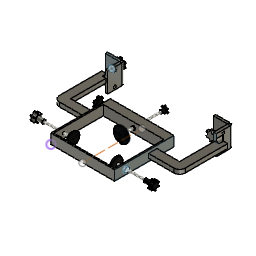
Wheelchair_Bracket (Autodesk Fusion 360 design; units mm, degrees)
Autodesk Fusion 360 part; units mm, degrees
note: some values were not read from the file. Chosen so that the rebuilt part matches the saved one: which face or edge a step refers to; how an offset face is resized.
sketch "Schizzo1" plane through (0, 0, 0) normal (0, 0, 1) x (1, 0, 0)
  line L0 (0, 0) -> (225, 0)
  line L1 (225, 0) -> (225, 210)
  line L2 (225, 210) -> (0, 210)
  line L3 (0, 210) -> (0, 0)
  line L4 (5, 180) -> (5, 5)
  line L5 (5, 5) -> (220, 5)
  line L6 (220, 5) -> (220, 180)
  line L7 (0, 150) -> (-75, 150)
  line L8 (0, 120) -> (-110, 120)
  line L9 (-110, 120) -> (-110, 290)
  line L10 (-110, 290) -> (-80, 290)
  line L11 (-80, 290) -> (-80, 150)
  line L12 (-80, 150) -> (-75, 150)
  line L13 (335, 120) -> (335, 290)
  line L14 (305, 290) -> (305, 150)
  line L15 (335, 290) -> (305, 290)
  line L16 (225, 120) -> (335, 120)
  line L17 (225, 150) -> (300, 150)
  line L18 (300, 150) -> (305, 150)
  line L19 (5, 180) -> (220, 180)
  dimension "d1" = 225
  dimension "d2" = 210
  dimension "d5" = 30
  dimension "d8" = 30
  constraint horizontal L0
  constraint vertical L1
  constraint horizontal L2
  constraint vertical L3
  constraint coincident L0.start L3.end
  constraint coincident L3 L7.start
  constraint perpendicular L3 L7
  constraint coincident L3 L8.start
  constraint perpendicular L3 L8
  constraint perpendicular L8 L9
  constraint perpendicular L9 L10
  constraint perpendicular L7 L11
  constraint perpendicular L11 L12
  constraint perpendicular L1 L19
  constraint parallel L3 L4
  constraint parallel L0 L5
  constraint parallel L1 L6
  measures "d1" distance of L0.start L0.end
  measures "d2" distance of L0.start L2.end
  measures "d5" distance of L7 L8
  measures "d8" distance of L2 L19
extrude "Estrusione1" add sketch "Schizzo1" along normal blind 35 contours L0 L1 L2 L3 makes body 1
extrude "Estrusione2" add sketch "Schizzo1" along normal blind 25 contours L3 L7 L8 L9 L10 L11 L12 | L1 L13 L14 L15 L16 L17 L18 bodies 1
extrude "Estrusione3" cut sketch "Schizzo1" along normal blind 10 contours L3 L7 L8 L9 L10 L11 L12 | L1 L13 L14 L15 L16 L17 L18 bodies 1
sketch "Schizzo2" plane through (0, 180, 0) normal (0, -1, 0) x (1, 0, 0)
  line L0 (5, 0) -> (220, 0)
  line L1 (220, 0) -> (220, 35)
  line L2 (220, 35) -> (5, 35)
  line L3 (5, 35) -> (5, 0)
sketch "Schizzo3" plane through (0, 210, 0) normal (0, 1, 0) x (-1, 0, 0)
  line L0 (-225, 0) -> (0, 0)
  line L1 (0, 0) -> (0, 35)
  line L2 (0, 35) -> (-225, 35)
  line L3 (-225, 35) -> (-225, 0)
  circle A0 centre (-112.5, 17.5615) radius 4
  dimension "d17" = 8
  dimension "d18" = 112.5
  measures "d17" diameter of A0
  measures "d18" distance of L3 A0.centre
extrude "Estrusione5" cut sketch "Schizzo3" along normal mid plane 100 contours A0 bodies 1
extrude "Estrusione8" add sketch "Schizzo3" along normal mid plane 140 separate body contours A0 makes body 2
thread "Filettatura2" "ISO Metric profile 8.0 M8x1.25 6g" major diameter 7.866 minor diameter 6.4455 pitch 1.25 angle 60 resizes the face on face at (108.5199, 256.6667, 17.1632) on bodies 2
sketch "Schizzo4" plane through (0, 280, 0) normal (0, 1, 0) x (-1, 0, 0)
  circle A0 centre (-112.5, 17.5615) radius 3.933
  circle A1 centre (-112.5, 17.5615) radius 6.5
  dimension "d29" = 13
  constraint concentric A0 A1
  measures "d29" diameter of A1
extrude "Estrusione9" add sketch "Schizzo4" along normal blind 8 contours A0 | A1 bodies 2
extrude "Estrusione10" add 1 faces at (106.8945, 280, 17.0432) along direction (0, -1, 0) blind 3 on bodies 2 bodies 2
sketch "Schizzo6" plane through (0, 288, 0) normal (0, 1, 0) x (-1, 0, 0)
  circle A0 centre (-112.5, 17.5615) radius 6.5
  circle A1 centre (-112.5, 17.5615) radius 12.5
  circle A2 centre (-125, 17.5615) radius 6.1387
  circle A3 centre (-118.75, 6.7362) radius 6.1387
  circle A4 centre (-106.25, 6.7362) radius 6.1387
  circle A5 centre (-100, 17.5615) radius 6.1387
  circle A6 centre (-106.25, 28.3868) radius 6.1387
  circle A7 centre (-118.75, 28.3868) radius 6.1387
  dimension "d38" = 25
  dimension "d40" = 360
  constraint concentric A0 A1
  constraint coincident A1 A2.centre
  measures "d38" diameter of A1
extrude "Estrusione12" add sketch "Schizzo6" along normal blind 6 contours A0 A2 A3 A4 A5 A6 A7 | A0 A1 A5 A6 | A0 A1 A4 A5 | A0 A1 A6 A7 | A0 A1 A3 A4 | A0 A1 A2 A7 | A0 A1 A2 A3 bodies 2
fillet "Raccordo3" radius 20 1 edges at (-110, 120, 17.5) on bodies 1
fillet "Raccordo4" radius 20 1 edges at (335, 120, 17.5) on bodies 1
sketch "Schizzo7" plane through (0, 0, 0) normal (0, 0, 1) x (1, 0, 0)
sketch "Schizzo8" plane through (0, 140, 0) normal (0, -1, 0) x (1, 0, 0)
  circle A0 centre (112.5, 17.5615) radius 3.933
  circle A1 centre (112.5, 17.5615) radius 25
  dimension "d51" = 50
  constraint concentric A0 A1
  measures "d51" diameter of A1
extrude "Estrusione13" add sketch "Schizzo8" along normal blind 5 draft 20 separate body makes body 3
sketch "Schizzo9" plane through (225, 0, 0) normal (1, 0, 0) x (0, 1, 0)
  line L0 (0, 0) -> (210, 0)
  line L1 (210, 0) -> (210, 35)
  line L2 (210, 35) -> (0, 35)
  line L3 (0, 35) -> (0, 0)
  line L4 (150, 10) -> (120, 10)
  line L5 (120, 10) -> (120, 25)
  line L6 (120, 25) -> (150, 25)
  line L7 (150, 25) -> (150, 10)
  circle A0 centre (40, 17.5) radius 4
  line L8 (0, 0) -> (210, 0)
  dimension "d54" = 8
  dimension "d55" = 40
  dimension "d56" = 17.5
  measures "d54" diameter of A0
  measures "d55" distance of L3 A0.centre
  measures "d56" distance of A0.centre L8
extrude "Estrusione15" add sketch "Schizzo9" along normal blind 80 separate body contours A0 makes body 4
extrude "Estrusione23" add sketch "Schizzo9" against normal blind 30 contours A0 bodies 4
thread "Filettatura4" "ISO Metric profile 8.0 M8x1.25 6g" major diameter 7.866 minor diameter 6.4455 pitch 1.25 angle 60 resizes the face on face at (278.3333, 43.995, 17.3006) on bodies 4
sketch "Schizzo13" plane through (195, 0, 0) normal (-1, 0, 0) x (0, -1, 0)
  circle A0 centre (-40, 17.5) radius 3.933
  circle A1 centre (-40, 17.5) radius 20
  dimension "d83" = 40
  constraint concentric A0 A1
  measures "d83" diameter of A1
extrude "Estrusione24" add sketch "Schizzo13" along normal blind 5 draft 25 separate body makes body 5
sketch "Schizzo14" plane through (305, 0, 0) normal (1, 0, 0) x (0, 1, 0)
  circle A0 centre (40, 17.5) radius 3.933
  circle A1 centre (40, 17.5) radius 7.5
  dimension "d86" = 15
  constraint concentric A0 A1
  measures "d86" diameter of A1
extrude "Estrusione25" add sketch "Schizzo14" along normal mid plane 20 bodies 4
extrude "Estrusione26" add 1 faces at (305, 38.9168, 16.3707) along direction (1, 0, 0) blind 10 on bodies 4 bodies 4
sketch "Schizzo15" plane through (0, 0, 0) normal (0, 0, 1) x (1, 0, 0)
sketch "Schizzo16" plane through (315, 0, 0) normal (1, 0, 0) x (0, 1, 0)
  circle A0 centre (40, 17.5) radius 7.5
  circle A1 centre (40, 17.5) radius 15
  circle A2 centre (25, 17.5) radius 6
  circle A3 centre (32.5, 4.5096) radius 6
  circle A4 centre (47.5, 4.5096) radius 6
  circle A5 centre (55, 17.5) radius 6
  circle A6 centre (47.5, 30.4904) radius 6
  circle A7 centre (32.5, 30.4904) radius 6
  dimension "d91" = 30
  dimension "d92" = 12
  dimension "d94" = 360
  constraint concentric A0 A1
  constraint coincident A1 A2.centre
  measures "d91" diameter of A1
  measures "d92" diameter of A2
extrude "Estrusione27" add sketch "Schizzo16" along normal blind 15 contours A0 | A1 A2 A3 A4 A5 A6 A7 bodies 4
sketch "Schizzo17" plane through (0, 0, 0) normal (0, 0, 1) x (1, 0, 0)
  line L0 (112.5, 0) -> (112.5, 210) construction
  dimension "d97" = 112.5
  constraint vertical L0
  measures "d97" distance of L0.start origin
ref_plane "Piano di lavoro1" through (115, 105, 17.5) normal (1, 0, 0) x (0, 1, 0)
mirror "Specchio1" about plane through (115, 105, 17.5) normal (1, 0, 0) of bodies 4 5 makes body 6 at (-31.6667, 43.9281, 17.304) makes body 7 at (40, 24.6676, 16.311)
sketch "Schizzo18" plane through (305, 0, 0) normal (-1, 0, 0) x (0, -1, 0)
  line L0 (-290, 10) -> (-150, 10)
  line L1 (-150, 10) -> (-150, 25)
  line L2 (-150, 25) -> (-290, 25)
  line L3 (-290, 25) -> (-290, 10)
  line L4 (-275, -20) -> (-325, -20)
  line L5 (-325, -20) -> (-325, 50)
  line L6 (-325, 50) -> (-275, 50)
  line L7 (-275, 50) -> (-275, -20)
  constraint horizontal L4
  constraint vertical L5
  constraint horizontal L6
  constraint vertical L7
extrude "Estrusione28" add sketch "Schizzo18" along normal blind 5 contours L0 L2 L3 L7 | L0 L2 L3 L4 L5 L6 L7 bodies 1
extrude "Estrusione29" add 1 faces at (305, 313.3333, 13.3333) along direction (1, 0, 0) blind 5 on bodies 1 bodies 1
sketch "Schizzo19" plane through (300, 0, 0) normal (-1, 0, 0) x (0, -1, 0)
  line L0 (-275, 50) -> (-325, 50)
  line L1 (-325, 50) -> (-325, -20)
  line L2 (-325, -20) -> (-275, -20)
  line L3 (-275, -20) -> (-275, 50)
  circle A0 centre (-300, -10) radius 5
  circle A1 centre (-300, 40) radius 5
  dimension "d104" = 10
  dimension "d105" = 10
  measures "d104" diameter of A0
  measures "d105" diameter of A1
extrude "Estrusione30" cut sketch "Schizzo19" against normal blind 35 contours A0 | A1 bodies 1
fillet "Raccordo5" radius 10 3 edges at (310, 282.5, 10) (310, 290, 17.5) (310, 282.5, 25) on bodies 1
sketch "Schizzo1 (2)" plane through (0, 275, 0) normal (0, -1, 0) x (1, 0, 0) in component "Component"
  line L0 (310, 50) -> (300, 50)
  line L1 (300, 50) -> (300, -20)
  line L2 (300, -20) -> (310, -20)
  line L3 (310, -20) -> (310, 0)
  arc A0 (320, 10) -> (310, 0) centre (320, 0) ccw
  line L4 (320, 10) -> (305, 10)
  line L5 (305, 10) -> (305, 25)
  line L6 (305, 25) -> (320, 25)
  arc A1 (310, 35) -> (320, 25) centre (320, 35) ccw
  line L7 (310, 35) -> (310, 50)
sketch "Schizzo3 (2)" plane through (0, 325, 0) normal (0, 1, 0) x (-1, 0, 0) in component "Component"
  line L0 (-310, -20) -> (-300, -20)
  line L1 (-300, -20) -> (-300, 50)
  line L2 (-300, 50) -> (-310, 50)
  line L3 (-310, 50) -> (-310, -20)
sketch "Schizzo20" plane through (0, 0, 0) normal (0, 0, 1) x (1, 0, 0)
  circle A0 centre (305, 329) radius 4
  line L0 (300, 325) -> (310, 325)
  dimension "d112" = 8
  constraint tangent A0 L0
  measures "d112" diameter of A0
extrude "Estrusione31" add sketch "Schizzo20" along normal blind 50 separate body makes body 8
extrude "Estrusione32" add 1 faces at (305.2524, 327.9512, 0) along direction (0, 0, -1) blind 20 on bodies 8 bodies 8 4 5 6 7 1
sketch "Schizzo21" plane through (0, 325, 0) normal (0, 1, 0) x (-1, 0, 0)
  line L0 (-300, -20) -> (-250, -20)
  line L1 (-250, -20) -> (-250, 50)
  line L2 (-250, 50) -> (-300, 50)
  line L3 (-300, 50) -> (-300, -20)
  constraint horizontal L0
  constraint vertical L1
  constraint horizontal L2
  constraint vertical L3
extrude "Estrusione33" add sketch "Schizzo21" along normal blind 5 separate body makes body 9
extrude "Estrusione36" add 1 faces at (283.3333, 330, 26.6667) along direction (0, 1, 0) blind 3 on bodies 9 bodies 9
sketch "Schizzo22" plane through (0, 333, 0) normal (0, 1, 0) x (-1, 0, 0)
  line L0 (-300, 50) -> (-300, -20)
  line L1 (-300, -20) -> (-250, -20)
  line L2 (-250, -20) -> (-250, 50)
  line L3 (-250, 50) -> (-300, 50)
  circle A0 centre (-275, 17.5) radius 4
  dimension "d129" = 8
  dimension "d130" = 25
  dimension "d131" = 32.5
  measures "d129" diameter of A0
  measures "d130" distance of L2 A0.centre
  measures "d131" distance of L3 A0.centre
extrude "Estrusione37" add sketch "Schizzo22" along normal blind 20 and the other way blind 25 contours A0 bodies 9
thread "Filettatura5" "ISO Metric profile 8.0 M8x1.25 6g" major diameter 7.866 minor diameter 6.4455 pitch 1.25 angle 60 resizes the face on face at (272.665, 313.6667, 20.7478) on bodies 9
thread "Filettatura6" "ISO Metric profile 8.0 M8x1.25 6g" major diameter 7.866 minor diameter 6.4455 pitch 1.25 angle 60 resizes the face on face at (272.665, 339.6667, 20.7478) on bodies 9
sketch "Schizzo24" plane through (0, 308, 0) normal (0, -1, 0) x (1, 0, 0)
  circle A0 centre (275, 17.5) radius 3.933
  circle A1 centre (275, 17.5) radius 7.5
  dimension "d137" = 15
  constraint concentric A0 A1
  measures "d137" diameter of A1
extrude "Estrusione38" add sketch "Schizzo24" along normal mid plane 20 bodies 9
extrude "Estrusione39" add 1 faces at (276.5445, 308, 16.6083) along direction (0, -1, 0) blind 10 on bodies 9 bodies 9
sketch "Schizzo25" plane through (0, 298, 0) normal (0, -1, 0) x (1, 0, 0)
  circle A0 centre (275, 17.5) radius 7.5
  circle A1 centre (275, 17.5) radius 17.5
  circle A2 centre (257.5, 17.5) radius 6
  circle A3 centre (266.25, 2.3446) radius 6
  circle A4 centre (283.75, 2.3446) radius 6
  circle A5 centre (292.5, 17.5) radius 6
  circle A6 centre (283.75, 32.6554) radius 6
  circle A7 centre (266.25, 32.6554) radius 6
  dimension "d142" = 35
  dimension "d143" = 12
  dimension "d145" = 360
  constraint concentric A0 A1
  constraint coincident A1 A2.centre
  measures "d142" diameter of A1
  measures "d143" diameter of A2
extrude "Estrusione40" add sketch "Schizzo25" along normal blind 8 contours A0 | A1 A2 A3 A4 A5 A6 A7 bodies 9
extrude "Estrusione41" cut 1 faces at (277.6423, 318, 11.7874) along direction (0, -1, 0) blind 10 on bodies 9 bodies 9
sketch "Schizzo26" plane through (0, 333, 0) normal (0, 1, 0) x (-1, 0, 0)
  circle A0 centre (-275, 17.5) radius 3.933
  line L0 (-300, 50) -> (-300, -20)
  line L1 (-300, -20) -> (-250, -20)
  line L2 (-250, -20) -> (-250, 50)
  line L3 (-250, 50) -> (-300, 50)
  line L4 (-268.0719, 17.4702) -> (-271.5101, 23.485)
  line L5 (-271.5101, 23.485) -> (-278.4383, 23.5148)
  line L6 (-278.4383, 23.5148) -> (-281.9281, 17.5298)
  line L7 (-281.9281, 17.5298) -> (-278.4899, 11.515)
  line L8 (-278.4899, 11.515) -> (-271.5617, 11.4852)
  line L9 (-271.5617, 11.4852) -> (-268.0719, 17.4702)
  point P0 (-275, 17.5)
  dimension "d150" = 6
  constraint coincident P0 A0.centre
  measures "d150" distance of P0 L9
extrude "Estrusione42" add sketch "Schizzo26" along normal blind 2 separate body contours L4 L5 L6 L7 L8 L9 makes body 10
sketch "Schizzo27" plane through (0, 180, 0) normal (0, -1, 0) x (1, 0, 0)
  circle A0 centre (112.5, 17.5615) radius 4
  line L0 (5, 0) -> (220, 0)
  line L1 (220, 0) -> (220, 35)
  line L2 (220, 35) -> (5, 35)
  line L3 (5, 35) -> (5, 0)
  line L4 (119.4226, 17.8407) -> (115.7195, 23.6962)
  line L5 (115.7195, 23.6962) -> (108.7969, 23.417)
  line L6 (108.7969, 23.417) -> (105.5774, 17.2822)
  line L7 (105.5774, 17.2822) -> (109.2805, 11.4267)
  line L8 (109.2805, 11.4267) -> (116.2031, 11.706)
  line L9 (116.2031, 11.706) -> (119.4226, 17.8407)
  point P0 (112.5, 17.5615)
  dimension "d153" = 6
  constraint coincident P0 A0.centre
  measures "d153" distance of P0 L9
extrude "Estrusione43" add sketch "Schizzo27" along normal blind 2 separate body contours L4 L5 L6 L7 L8 L9 makes body 11
sketch "Schizzo28" plane through (225, 0, 0) normal (1, 0, 0) x (0, 1, 0)
  line L0 (0, 0) -> (210, 0)
  line L1 (210, 0) -> (210, 35)
  line L2 (210, 35) -> (0, 35)
  line L3 (0, 35) -> (0, 0)
  line L4 (150, 10) -> (120, 10)
  line L5 (120, 10) -> (120, 25)
  line L6 (120, 25) -> (150, 25)
  line L7 (150, 25) -> (150, 10)
  line L8 (41.2349, 25.5706) -> (34.8128, 23.9335)
  line L9 (34.8128, 23.9335) -> (31.4294, 18.2349)
  line L10 (31.4294, 18.2349) -> (33.0665, 11.8128)
  line L11 (33.0665, 11.8128) -> (38.7651, 8.4294)
  line L12 (38.7651, 8.4294) -> (45.1872, 10.0665)
  line L13 (45.1872, 10.0665) -> (48.5706, 15.7651)
  line L14 (48.5706, 15.7651) -> (46.9335, 22.1872)
  line L15 (46.9335, 22.1872) -> (41.2349, 25.5706)
  point P0 (40, 17)
  dimension "d156" = 8
  measures "d156" distance of P0 L15
extrude "Estrusione44" add sketch "Schizzo28" along normal blind 4 separate body contours L8 L9 L10 L11 L12 L13 L14 L15 makes body 12
mirror "Specchio2" about plane through (115, 105, 17.5) normal (1, 0, 0) of bodies 12 makes body 13
mirror "Specchio3" about plane through (115, 105, 17.5) normal (1, 0, 0) of bodies 12 makes body 14
mirror "Specchio4" about plane through (115, 105, 17.5) normal (1, 0, 0) of bodies 12 makes body 15
extrude "Estrusione45" add 1 faces at (5, 39.5884, 14.1431) along direction (-1, 0, 0) blind 10 on bodies 15 bodies 15 7 11 12 6 8 13 14
sketch "Schizzo29" plane through (0, 0, 0) normal (0, 0, 1) x (1, 0, 0)
sketch "Schizzo30" plane through (0, 0, 0) normal (-1, 0, 0) x (0, -1, 0)
  line L0 (-41.2349, 25.5706) -> (-34.8128, 23.9335)
  line L1 (-34.8128, 23.9335) -> (-31.4294, 18.2349)
  line L2 (-31.4294, 18.2349) -> (-33.0665, 11.8128)
  line L3 (-33.0665, 11.8128) -> (-38.7651, 8.4294)
  line L4 (-38.7651, 8.4294) -> (-45.1872, 10.0665)
  line L5 (-45.1872, 10.0665) -> (-48.5706, 15.7651)
  line L6 (-48.5706, 15.7651) -> (-46.9335, 22.1872)
  line L7 (-46.9335, 22.1872) -> (-41.2349, 25.5706)
  line L8 (-120, 10) -> (-150, 10)
  line L9 (-150, 10) -> (-150, 25)
  line L10 (-150, 25) -> (-120, 25)
  line L11 (-120, 25) -> (-120, 10)
  line L12 (-210, 0) -> (0, 0)
  line L13 (0, 0) -> (0, 35)
  line L14 (0, 35) -> (-210, 35)
  line L15 (-210, 35) -> (-210, 0)
  circle A0 centre (-194.5679, 17.5) radius 4
  dimension "d169" = 8
  dimension "d170" = 17.5
  measures "d169" diameter of A0
  measures "d170" distance of L14 A0.centre
extrude "Estrusione46" add sketch "Schizzo30" along normal blind 20 and the other way blind 0 separate body contours A0 makes body 16
thread "Filettatura7" "ISO Metric profile 8.0 M8x1.25 6g" major diameter 7.866 minor diameter 6.4455 pitch 1.25 angle 60 resizes the face on face at (-13.3333, 197.6321, 20.0712) on bodies 16
sketch "Schizzo31" plane through (0, 0, 0) normal (-1, 0, 0) x (0, -1, 0)
  line L0 (-41.2349, 25.5706) -> (-34.8128, 23.9335)
  line L1 (-34.8128, 23.9335) -> (-31.4294, 18.2349)
  line L2 (-31.4294, 18.2349) -> (-33.0665, 11.8128)
  line L3 (-33.0665, 11.8128) -> (-38.7651, 8.4294)
  line L4 (-38.7651, 8.4294) -> (-45.1872, 10.0665)
  line L5 (-45.1872, 10.0665) -> (-48.5706, 15.7651)
  line L6 (-48.5706, 15.7651) -> (-46.9335, 22.1872)
  line L7 (-46.9335, 22.1872) -> (-41.2349, 25.5706)
  line L8 (-120, 10) -> (-150, 10)
  line L9 (-150, 10) -> (-150, 25)
  line L10 (-150, 25) -> (-120, 25)
  line L11 (-120, 25) -> (-120, 10)
  line L12 (-210, 0) -> (0, 0)
  line L13 (0, 0) -> (0, 35)
  line L14 (0, 35) -> (-210, 35)
  line L15 (-210, 35) -> (-210, 0)
  line L16 (-184.6108, 15.2535) -> (-190.0249, 24.1241)
  line L17 (-190.0249, 24.1241) -> (-200.4141, 23.8706)
  line L18 (-200.4141, 23.8706) -> (-205.3892, 14.7465)
  line L19 (-205.3892, 14.7465) -> (-199.9751, 5.8759)
  line L20 (-199.9751, 5.8759) -> (-189.5859, 6.1294)
  line L21 (-189.5859, 6.1294) -> (-184.6108, 15.2535)
  point P0 (-195, 15)
  dimension "d175" = 9
  measures "d175" distance of P0 L21
extrude "Estrusione47" add sketch "Schizzo31" along normal blind 5 separate body contours L16 L17 L18 L19 L20 L21 makes body 17
sketch "Schizzo32" plane through (-20, 0, 0) normal (-1, 0, 0) x (0, -1, 0)
  circle A0 centre (-194.5679, 17.5) radius 3.933
  circle A1 centre (-194.5679, 17.5) radius 7.5
  dimension "d178" = 15
  constraint concentric A0 A1
  measures "d178" diameter of A1
extrude "Estrusione48" add sketch "Schizzo32" along normal blind 5 and the other way blind 5 contours A0 | A1 bodies 16
sketch "Schizzo33" plane through (-25, 0, 0) normal (-1, 0, 0) x (0, -1, 0)
  circle A0 centre (-194.5679, 17.5) radius 7.5
  circle A1 centre (-194.5679, 17.5) radius 17.5
  circle A2 centre (-212.0679, 17.5) radius 5
  circle A3 centre (-203.3179, 2.3446) radius 5
  circle A4 centre (-185.8179, 2.3446) radius 5
  circle A5 centre (-177.0679, 17.5) radius 5
  circle A6 centre (-185.8179, 32.6554) radius 5
  circle A7 centre (-203.3179, 32.6554) radius 5
  dimension "d183" = 35
  dimension "d184" = 10
  dimension "d186" = 360
  constraint concentric A0 A1
  constraint coincident A1 A2.centre
  measures "d183" diameter of A1
  measures "d184" diameter of A2
extrude "Estrusione49" add sketch "Schizzo33" along normal blind 5 contours A0 | A1 A2 A3 A4 A5 A6 A7 bodies 16
sketch "Schizzo34" plane through (-80, 0, 0) normal (1, 0, 0) x (0, 1, 0)
  line L0 (150, 10) -> (290, 10)
  line L1 (290, 10) -> (290, 25)
  line L2 (290, 25) -> (150, 25)
  line L3 (150, 25) -> (150, 10)
  line L4 (275, 50) -> (325, 50)
  line L5 (325, 50) -> (325, -20)
  line L6 (325, -20) -> (275, -20)
  line L7 (275, -20) -> (275, 50)
  dimension "d189" = 50
  dimension "d190" = 70
  constraint horizontal L4
  constraint vertical L5
  constraint horizontal L6
  constraint vertical L7
  measures "d189" distance of L4.start L4.end
  measures "d190" distance of L4.start L6.end
extrude "Estrusione51" add sketch "Schizzo34" along normal blind 5 separate body contours L0 L1 L2 L7 | L0 L1 L2 L4 L5 L6 L7 makes body 18
extrude "Estrusione53" add sketch "Schizzo34" against normal blind 3 contours L0 L1 L2 L4 L5 L6 L7 bodies 18 16 17 15
extrude "Estrusione54" add 1 faces at (-75, 291.6667, 26.6667) along direction (1, 0, 0) blind 1 on bodies 18 bodies 18
fillet "Raccordo6" radius 10 3 edges at (-83, 282.5, 25) (-83, 290, 17.5) (-83, 282.5, 10) on bodies 18
mirror "Specchio6" about plane through (115, 105, 17.5) normal (1, 0, 0) of "Estrusione30"
sketch "Schizzo35" plane through (0, 0, 0) normal (0, 0, 1) x (1, 0, 0)
  circle A0 centre (-78.5392, 329) radius 4
  line L0 (-83, 325) -> (-74, 325)
  dimension "d205" = 8
  constraint tangent A0 L0
  measures "d205" diameter of A0
extrude "Estrusione55" add sketch "Schizzo35" along normal blind 50 and the other way blind 20 separate body makes body 19
thread "Filettatura8" "ISO Metric profile 8.0 M8x1.25 6g" major diameter 7.866 minor diameter 6.4455 pitch 1.25 angle 60 resizes the face on face at (-74.6519, 328.057, 33.3333) on bodies 19
sketch "Schizzo36" plane through (0, 325, 0) normal (0, 1, 0) x (-1, 0, 0)
  line L0 (83, 50) -> (74, 50)
  line L1 (74, 50) -> (74, -20)
  line L2 (74, -20) -> (83, -20)
  line L3 (83, -20) -> (83, 50)
  line L4 (83, -20) -> (133, -20)
  line L5 (133, -20) -> (133, 50)
  line L6 (133, 50) -> (83, 50)
  line L7 (83, 50) -> (83, -20)
  dimension "d210" = 50
  dimension "d211" = 70
  constraint horizontal L4
  constraint vertical L5
  constraint horizontal L6
  constraint vertical L7
  constraint coincident L2.end L3.start
  measures "d210" distance of L2.end L4.end
  measures "d211" distance of L2.end L0.start
extrude "Estrusione56" add sketch "Schizzo36" along normal blind 8 separate body contours L3 L4 L5 L6 L7 makes body 20
sketch "Schizzo37" plane through (0, 333, 0) normal (0, 1, 0) x (-1, 0, 0)
  line L0 (83, 50) -> (83, -20)
  line L1 (83, -20) -> (133, -20)
  line L2 (133, -20) -> (133, 50)
  line L3 (133, 50) -> (83, 50)
  circle A0 centre (110.5, 15) radius 4
  dimension "d214" = 8
  dimension "d215" = 35
  dimension "d216" = 22.5
  measures "d214" diameter of A0
  measures "d215" distance of L3 A0.centre
  measures "d216" distance of L2 A0.centre
extrude "Estrusione57" add sketch "Schizzo37" along normal blind 20 and the other way blind 30 contours A0 bodies 20
thread "Filettatura9" "ISO Metric profile 8.0 M8x1.25 6g" major diameter 7.866 minor diameter 6.4455 pitch 1.25 angle 60 resizes the face on face at (-114.4801, 317.6667, 14.6017) on bodies 20
thread "Filettatura10" "ISO Metric profile 8.0 M8x1.25 6g" major diameter 7.866 minor diameter 6.4455 pitch 1.25 angle 60 resizes the face on face at (-114.4801, 346.3333, 15.3983) on bodies 20
extrude "Estrusione58" cut 1 faces at (-111.3174, 303, 17.1626) along direction (0, 1, 0) blind 10 on bodies 20 bodies 20
sketch "Schizzo38" plane through (0, 325, 0) normal (0, -1, 0) x (1, 0, 0)
  circle A0 centre (-110.5, 15) radius 3.933
  line L0 (-83, -20) -> (-83, 50)
  line L1 (-83, 50) -> (-133, 50)
  line L2 (-133, 50) -> (-133, -20)
  line L3 (-133, -20) -> (-83, -20)
  point P0 (-110.5, 11.067)
  constraint coincident A0 P0
sketch "Schizzo39" plane through (0, 325, 0) normal (0, -1, 0) x (1, 0, 0)
  line L0 (-104.2905, 7.7381) -> (-100.8563, 16.3136)
  line L1 (-100.8563, 16.3136) -> (-106.5658, 23.5755)
  line L2 (-106.5658, 23.5755) -> (-115.7095, 22.2619)
  line L3 (-115.7095, 22.2619) -> (-119.1437, 13.6864)
  line L4 (-119.1437, 13.6864) -> (-113.4342, 6.4245)
  line L5 (-113.4342, 6.4245) -> (-104.2905, 7.7381)
  point P0 (-110, 15)
  dimension "d224" = 8
  measures "d224" distance of P0 L5
extrude "Estrusione59" add sketch "Schizzo39" along normal blind 3 separate body makes body 21
sketch "Schizzo43" plane through (0, 353, 0) normal (0, 1, 0) x (-1, 0, 0)
  circle A0 centre (110.5, 15) radius 3.933
  circle A1 centre (110.5, 15) radius 7.5
  dimension "d233" = 15
  constraint concentric A0 A1
  measures "d233" diameter of A1
extrude "Estrusione62" add sketch "Schizzo43" along normal blind 2 and the other way blind 2 separate body contours A0 | A1 makes body 22
sketch "Schizzo44" plane through (0, 355, 0) normal (0, 1, 0) x (-1, 0, 0)
  circle A0 centre (110.5, 15) radius 7.5
  circle A1 centre (110.5, 15) radius 17.5
  circle A2 centre (93, 15) radius 5
  circle A3 centre (101.75, -0.1554) radius 5
  circle A4 centre (119.25, -0.1554) radius 5
  circle A5 centre (128, 15) radius 5
  circle A6 centre (119.25, 30.1554) radius 5
  circle A7 centre (101.75, 30.1554) radius 5
  dimension "d238" = 35
  dimension "d239" = 10
  dimension "d241" = 360
  constraint concentric A0 A1
  constraint coincident A1 A2.centre
  measures "d238" diameter of A1
  measures "d239" diameter of A2
extrude "Estrusione63" add sketch "Schizzo44" along normal blind 5 separate body contours A0 | A1 A2 A3 A4 A5 A6 A7 makes body 23
sketch "Schizzo42" plane through (0, 333, 0) normal (0, 1, 0) x (-1, 0, 0)
  circle A0 centre (110.5737, 15.0037) radius 7.5
  dimension "d228" = 15
  measures "d228" diameter of A0
extrude "Estrusione61" [rolled back] along distance 17 taper angle 0
extrude "Estrusione60" [rolled back] along distance 22 taper angle 0
sketch "Schizzo40" plane through (0, 325, 0) normal (0, -1, 0) x (1, 0, 0)
sketch "Schizzo41" plane through (0, 325, 0) normal (0, -1, 0) x (1, 0, 0)
  circle A0 centre (-110.5382, 14.8984) radius 7.5
  dimension "d227" = 15
  measures "d227" diameter of A0
extrude "Estrusione52" [rolled back] along distance 5 taper angle 0
extrude "Estrusione50" [rolled back] along distance 5 taper angle 0
mirror "Specchio5" [rolled back] mirror stitch tolerance 0.1
sketch "Schizzo23" plane through (0, 308, 0) normal (0, -1, 0) x (1, 0, 0)
  circle A0 centre (275, 17.5) radius 3.933
  circle A1 centre (275, 17.5) radius 17.5
  dimension "d136" = 35
  constraint concentric A0 A1
  measures "d136" diameter of A1
extrude "Estrusione35" [rolled back] along distance 5 taper angle 0
extrude "Estrusione34" [rolled back] along distance 5 taper angle 0
sketch "Schizzo2 (2)" plane through (0, 325, 0) normal (0, 1, 0) x (-1, 0, 0) in component "Component"
  line L0 (-310, -20) -> (-300, -20)
  line L1 (-300, -20) -> (-300, 50)
  line L2 (-300, 50) -> (-310, 50)
  line L3 (-310, 50) -> (-310, -20)
  line L4 (-310, -20) -> (-250, -20)
  line L5 (-250, -20) -> (-250, 50)
  line L6 (-250, 50) -> (-310, 50)
  line L7 (-310, 50) -> (-310, -20)
  constraint horizontal L4
  constraint vertical L5
  constraint horizontal L6
  constraint vertical L7
  constraint coincident L0.start L3.end
extrude "Estrusione1'" [rolled back] along distance 5 taper angle 0 in component "Component"
extrude "Estrusione16" [rolled back] along distance -25 taper angle 0
extrude "Estrusione17" [rolled back] along distance 20 taper angle 0
thread "Filettatura3" [rolled back]
sketch "Schizzo10" plane through (200, 0, 0) normal (-1, 0, 0) x (0, -1, 0)
  circle A0 centre (-40, 17.5) radius 3.933
  circle A1 centre (-40, 17.5) radius 20
  dimension "d65" = 40
  constraint concentric A0 A1
  measures "d65" diameter of A1
extrude "Estrusione18" [rolled back] along distance 5 taper angle 25
sketch "Schizzo11" plane through (305, 0, 0) normal (1, 0, 0) x (0, 1, 0)
  circle A0 centre (40, 17.5) radius 3.933
  circle A1 centre (40, 17.5) radius 7.5
  dimension "d68" = 15
  constraint concentric A0 A1
  measures "d68" diameter of A1
extrude "Estrusione19" [rolled back] along distance 5 taper angle 0
extrude "Estrusione20" [rolled back] along distance 5 taper angle 0
sketch "Schizzo12" plane through (310, 0, 0) normal (1, 0, 0) x (0, 1, 0)
  circle A0 centre (40, 17.5) radius 7.5
  circle A1 centre (40, 17.5) radius 17.5
  circle A2 centre (22.5, 17.5) radius 6
  circle A3 centre (31.25, 2.3446) radius 6
  circle A4 centre (48.75, 2.3446) radius 6
  circle A5 centre (57.5, 17.5) radius 6
  circle A6 centre (48.75, 32.6554) radius 6
  circle A7 centre (31.25, 32.6554) radius 6
  dimension "d73" = 35
  dimension "d74" = 12
  dimension "d76" = 360
  constraint concentric A0 A1
  constraint coincident A1 A2.centre
  measures "d73" diameter of A1
  measures "d74" diameter of A2
extrude "Estrusione22" [rolled back] along distance 10 taper angle 0
extrude "Estrusione21" [rolled back] along distance 10 taper angle 0
extrude "Estrusione14" [rolled back] along distance 70 taper angle 0
fillet "Raccordo1" [rolled back] radius 3.5
fillet "Raccordo2" [rolled back] radius 6.5
sketch "Schizzo5" plane through (0, 288, 0) normal (0, 1, 0) x (-1, 0, 0)
  circle A0 centre (-118.75, 28.3868) radius 8.5545
  circle A1 centre (-127.3042, 28.4578) radius 8.3306
  circle A2 centre (-125.9846, 23.8217) radius 8.3306
  circle A3 centre (-122.3681, 20.6351) radius 8.3306
  circle A4 centre (-117.6029, 19.9095) radius 8.3306
  circle A5 centre (-113.2018, 21.8755) radius 8.3306
  circle A6 centre (-110.5623, 25.9087) radius 8.3306
  circle A7 centre (-110.5223, 30.7287) radius 8.3306
  circle A8 centre (-113.0945, 34.8052) radius 8.3306
  circle A9 centre (-117.4624, 36.8439) radius 8.3306
  circle A10 centre (-122.239, 36.1975) radius 8.3306
  circle A11 centre (-125.9079, 33.0713) radius 8.3306
  arc A12 (-116.5246, 22.6656) -> (-114.908, 23.599) centre (-118.75, 28.3868) ccw
  arc A13 (-114.908, 23.599) -> (-116.5246, 22.6656) centre (-112.5, 17.5615) ccw
  arc A14 (-106.0674, 18.4948) -> (-106.0674, 16.6281) centre (-100, 17.5615) ccw
  arc A15 (-106.0674, 16.6281) -> (-106.0674, 18.4948) centre (-112.5, 17.5615) ccw
  arc A16 (-108.4754, 12.4573) -> (-110.092, 11.524) centre (-106.25, 6.7362) ccw
  arc A17 (-110.092, 11.524) -> (-108.4754, 12.4573) centre (-112.5, 17.5615) ccw
  arc A18 (-110.092, 23.599) -> (-108.4754, 22.6656) centre (-106.25, 28.3868) ccw
  arc A19 (-108.4754, 22.6656) -> (-110.092, 23.599) centre (-112.5, 17.5615) ccw
  dimension "d35" = 360
  constraint concentric A0 A12
  constraint coincident A0 A1.centre
extrude "Estrusione11" [rolled back] along distance 3 taper angle 0
extrude "Estrusione6" [rolled back] along distance 60 taper angle 0
extrude "Estrusione7" [rolled back] along distance -30 taper angle 0
thread "Filettatura1" [rolled back]
extrude "Estrusione4" [rolled back] along distance 70 taper angle 0
component "Component" placed x (1, 0, 0) y (0, 0, -1) z (0, 1, 0) at (-5, 350, 340)
